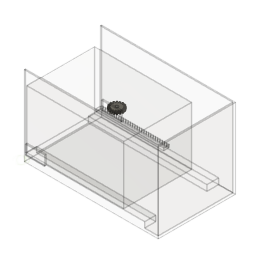
g25_gearmechanism_prototype (Autodesk Fusion 360 design; units mm, degrees)
part number: 2026-04-13-13-34-47-788
part number: 2026-04-13-16-24-35-810
part number: 2026-04-13-16-24-42-049
part number: 2026-04-13-16-24-44-900
Autodesk Fusion 360 part; units mm, degrees
sketch "AA_Sketch" plane through (0, 0, 0) normal (0, 0, 1) x (1, 0, 0)
  line L0 (0, 0) -> (283, 0)
  line L1 (283, 0) -> (283, 160)
  line L2 (283, 160) -> (0, 160)
  line L3 (0, 160) -> (0, 0)
  dimension "d1" = 283
  dimension "d2" = 160
  measures "d1" horizontal distance of L0.start L0.end
  measures "d2" vertical distance of L0.end L1.end
extrude "Extrude1" add sketch "AA_Sketch" along normal blind 165 makes body 1
shell "Shell1" thickness 3 removed faces 1 at (94.3333, 53.3333, 165) on bodies 1
sketch "Sketch2" plane through (0, 0, 3) normal (0, 0, 1) x (-1, 0, 0)
  line L0 (-3, -157) -> (-3, -3)
  line L1 (-3, -3) -> (-280, -3)
  line L2 (-280, -3) -> (-280, -157)
  line L3 (-280, -157) -> (-3, -157)
sketch "AA_Sketch (1)" plane through (0, 0, 0) normal (0, 0, 1) x (1, 0, 0)
  line L0 (0, 0) -> (200, 0)
  line L1 (200, 0) -> (200, 140)
  line L2 (200, 140) -> (0, 140)
  line L3 (0, 140) -> (0, 0)
  dimension "d6" = 200
  dimension "d7" = 140
  measures "d6" horizontal distance of L0.start L0.end
  measures "d7" vertical distance of L0.end L1.end
extrude "Extrude2" add sketch "AA_Sketch (1)" along normal blind 120 separate body makes body 2
move_body "Move1" bodies 2 to x (1, 0, 0) y (0, 1, 0) z (0, 0, 1) at (48.081, 9.2189, 0)
sketch "Sketch5" plane through (0, 3, 0) normal (0, 1, 0) x (-1, 0, 0)
  line L0 (-280, 3) -> (-3, 3)
  line L1 (-3, 3) -> (-3, 165)
  line L2 (-3, 165) -> (-280, 165)
  line L3 (-280, 165) -> (-280, 3)
sketch "AA_Sketch (2)" plane through (0, 0, 0) normal (0, 0, 1) x (1, 0, 0)
  line L0 (0, 0) -> (250, 0)
  line L1 (250, 0) -> (250, 5)
  line L2 (250, 5) -> (0, 5)
  line L3 (0, 5) -> (0, 0)
  dimension "d16" = 250
  dimension "d17" = 5
  measures "d16" horizontal distance of L0.start L0.end
  measures "d17" vertical distance of L0.end L1.end
sketch "AA_Sketch (2) (2)" plane through (0, 0, 0) normal (0, 0, 1) x (1, 0, 0)
  line L0 (0, 0) -> (250, 0)
  line L1 (250, 0) -> (250, 25)
  line L2 (250, 25) -> (0, 25)
  line L3 (0, 25) -> (0, 0)
  dimension "d10" = 250
  dimension "d11" = 25
  measures "d10" horizontal distance of L0.start L0.end
  measures "d11" vertical distance of L0.end L1.end
extrude "Extrude3" add sketch "AA_Sketch (2) (2)" along normal blind 7 separate body makes body 3
extrude "Extrude4" add 1 faces at (83.3333, 16.6667, 7) along direction (0, 0, 1) blind 7 on bodies 3 bodies 3
move_body "Move2" bodies 3 to x (1, 0, 0) y (0, 1, 0) z (0, 0, 1) at (1.9978, 0.899, 0.4525)
copy_body "CopyPasteBodies1" bodies 3 makes body 4
move_body "Move3" bodies 3 to x (1, 0, 0) y (0, 1, 0) z (0, 0, 1) at (-0.1358, 112.2274, 0)
move_body "Move4" bodies 3 to x (1, 0, 0) y (0, 1, 0) z (0, 0, 1) at (-1.6414, 34.1917, 0)
move_body "Move5" bodies 3 to x (1, 0, 0) y (0, 1, 0) z (0, 0, 1) at (0.433, 1.9595, 0)
move_face "MoveFace1" by (10.1391, 1.7367, 0) 1 faces at (83.9869, 165.9443, 14.4525) on bodies 3
move_body "Move6" bodies 2 to x (1, 0, 0) y (0, 1, 0) z (0, 0, 1) at (0, 1.2677, 9.5453)
move_body "Move7" bodies 2 to x (1, 0, 0) y (0, 1, 0) z (0, 0, 1) at (0, 0, 5.0574)
sketch "Base Circle" plane through (0, 0, 0) normal (0, 0, 1) x (1, 0, 0)
  circle A0 centre (0, 0) radius 10.2645
  circle A1 centre (0, 0) radius 3
extrude "Extrude6" add sketch "Base Circle" along normal blind 5 separate body makes body 5
sketch "Gear Tooth" plane through (0, 0, 0) normal (0, 0, 1) x (1, 0, 0)
  spline S0 degree 5 poles (11.2043, -1.2724) (11.2108, -1.2731) (11.2238, -1.2744) (11.2433, -1.2758) (11.2694, -1.2766) (11.3021, -1.2761) (11.3349, -1.2745) (11.3678, -1.2724) (11.4006, -1.2698) (11.4335, -1.267) (11.4664, -1.264) (11.4994, -1.2606) (11.5323, -1.2568) (11.5653, -1.2525) (11.5983, -1.2477) (11.6313, -1.2424) (11.6643, -1.2367) (11.6973, -1.2306) (11.7303, -1.2242) (11.7633, -1.2176) (11.7964, -1.2107) (11.8294, -1.2034) (11.8624, -1.1959) (11.8954, -1.188) (11.9285, -1.1798) (11.9615, -1.1713) (11.9945, -1.1625) (12.0275, -1.1534) (12.0605, -1.1441) (12.0935, -1.1345) (12.1265, -1.1246) (12.1594, -1.1145) (12.1924, -1.1041) (12.2253, -1.0934) (12.2583, -1.0825) (12.2912, -1.0713) (12.3241, -1.0599) (12.3569, -1.0482) (12.3898, -1.0363) (12.4226, -1.0241) (12.4555, -1.0117) (12.4883, -0.9991) (12.521, -0.9862) (12.5538, -0.9731) (12.5865, -0.9597) (12.6192, -0.9462) (12.6519, -0.9324) (12.6846, -0.9184) (12.7172, -0.9041) (12.7498, -0.8897) (12.7824, -0.875) (12.815, -0.8601) (12.8475, -0.845) (12.88, -0.8296) (12.9125, -0.8141) (12.9449, -0.7983) (12.9773, -0.7823) (13.0097, -0.7662) (13.042, -0.7498) (13.0743, -0.7332) (13.1066, -0.7164) (13.1388, -0.6994) (13.171, -0.6822) (13.2031, -0.6648) (13.2353, -0.6472) (13.2673, -0.6294) (13.2994, -0.6114) (13.3314, -0.5931) (13.3633, -0.5747) (13.3953, -0.5562) (13.4271, -0.5374) (13.4526, -0.5222) (13.4717, -0.5107) (13.4844, -0.503) (13.4908, -0.4992) knots 0 0 0 0 0 0 0.01428571 0.02857143 0.04285714 0.05714286 0.07142857 0.08571429 0.1 0.11428571 0.12857143 0.14285714 0.15714286 0.17142857 0.18571429 0.2 0.21428571 0.22857143 0.24285714 0.25714286 0.27142857 0.28571429 0.3 0.31428571 0.32857143 0.34285714 0.35714286 0.37142857 0.38571429 0.4 0.41428571 0.42857143 0.44285714 0.45714286 0.47142857 0.48571429 0.5 0.51428571 0.52857143 0.54285714 0.55714286 0.57142857 0.58571429 0.6 0.61428571 0.62857143 0.64285714 0.65714286 0.67142857 0.68571429 0.7 0.71428571 0.72857143 0.74285714 0.75714286 0.77142857 0.78571429 0.8 0.81428571 0.82857143 0.84285714 0.85714286 0.87142857 0.88571429 0.9 0.91428571 0.92857143 0.94285714 0.95714286 0.97142857 0.98571429 1 1 1 1 1 1
  spline S1 degree 5 poles (11.2043, 1.2724) (11.2108, 1.2731) (11.2238, 1.2744) (11.2433, 1.2758) (11.2694, 1.2766) (11.3021, 1.2761) (11.3349, 1.2745) (11.3678, 1.2724) (11.4006, 1.2698) (11.4335, 1.267) (11.4664, 1.264) (11.4994, 1.2606) (11.5323, 1.2568) (11.5653, 1.2525) (11.5983, 1.2477) (11.6313, 1.2424) (11.6643, 1.2367) (11.6973, 1.2306) (11.7303, 1.2242) (11.7633, 1.2176) (11.7964, 1.2107) (11.8294, 1.2034) (11.8624, 1.1959) (11.8954, 1.188) (11.9285, 1.1798) (11.9615, 1.1713) (11.9945, 1.1625) (12.0275, 1.1534) (12.0605, 1.1441) (12.0935, 1.1345) (12.1265, 1.1246) (12.1594, 1.1145) (12.1924, 1.1041) (12.2253, 1.0934) (12.2583, 1.0825) (12.2912, 1.0713) (12.3241, 1.0599) (12.3569, 1.0482) (12.3898, 1.0363) (12.4226, 1.0241) (12.4555, 1.0117) (12.4883, 0.9991) (12.521, 0.9862) (12.5538, 0.9731) (12.5865, 0.9597) (12.6192, 0.9462) (12.6519, 0.9324) (12.6846, 0.9184) (12.7172, 0.9041) (12.7498, 0.8897) (12.7824, 0.875) (12.815, 0.8601) (12.8475, 0.845) (12.88, 0.8296) (12.9125, 0.8141) (12.9449, 0.7983) (12.9773, 0.7823) (13.0097, 0.7662) (13.042, 0.7498) (13.0743, 0.7332) (13.1066, 0.7164) (13.1388, 0.6994) (13.171, 0.6822) (13.2031, 0.6648) (13.2353, 0.6472) (13.2673, 0.6294) (13.2994, 0.6114) (13.3314, 0.5931) (13.3633, 0.5747) (13.3953, 0.5562) (13.4271, 0.5374) (13.4526, 0.5222) (13.4717, 0.5107) (13.4844, 0.503) (13.4908, 0.4992) knots 0 0 0 0 0 0 0.01428571 0.02857143 0.04285714 0.05714286 0.07142857 0.08571429 0.1 0.11428571 0.12857143 0.14285714 0.15714286 0.17142857 0.18571429 0.2 0.21428571 0.22857143 0.24285714 0.25714286 0.27142857 0.28571429 0.3 0.31428571 0.32857143 0.34285714 0.35714286 0.37142857 0.38571429 0.4 0.41428571 0.42857143 0.44285714 0.45714286 0.47142857 0.48571429 0.5 0.51428571 0.52857143 0.54285714 0.55714286 0.57142857 0.58571429 0.6 0.61428571 0.62857143 0.64285714 0.65714286 0.67142857 0.68571429 0.7 0.71428571 0.72857143 0.74285714 0.75714286 0.77142857 0.78571429 0.8 0.81428571 0.82857143 0.84285714 0.85714286 0.87142857 0.88571429 0.9 0.91428571 0.92857143 0.94285714 0.95714286 0.97142857 0.98571429 1 1 1 1 1 1
  arc A0 (13.4908, -0.4992) -> (13.4908, 0.4992) centre (0, 0) ccw
  line L0 (10.189, -1.1571) -> (11.2043, -1.2724)
  line L1 (10.189, 1.1571) -> (11.2043, 1.2724)
  line L2 (10.189, -1.1571) -> (10.189, 1.1571)
  point P0 (11.3641, -1.2725)
  point P1 (11.5256, -1.2575)
  point P2 (11.688, -1.2323)
  point P3 (11.8512, -1.1984)
  point P4 (12.0149, -1.1569)
  point P5 (12.179, -1.1083)
  point P6 (12.3433, -1.053)
  point P7 (12.5078, -0.9914)
  point P8 (12.6722, -0.9237)
  point P9 (12.8365, -0.85)
  point P10 (13.0007, -0.7706)
  point P11 (13.1645, -0.6856)
  point P12 (13.3279, -0.5951)
  point P13 (11.3641, 1.2725)
  point P14 (11.5256, 1.2575)
  point P15 (11.688, 1.2323)
  point P16 (11.8512, 1.1984)
  point P17 (12.0149, 1.1569)
  point P18 (12.179, 1.1083)
  point P19 (12.3433, 1.053)
  point P20 (12.5078, 0.9914)
  point P21 (12.6722, 0.9237)
  point P22 (12.8365, 0.85)
  point P23 (13.0007, 0.7706)
  point P24 (13.1645, 0.6856)
  point P25 (13.3279, 0.5951)
extrude "Extrude7" add sketch "Gear Tooth" along normal blind 5 bodies 5
fillet "Fillet1" radius 0.5 2 edges at (10.1989, -1.1582, 2.5) (10.1989, 1.1582, 2.5) on bodies 5
pattern_circular "C-Pattern1" count 16 over 360 about axis through (0, 0, 0) along (0, 0, 1) of "Extrude7", "Fillet1"
sketch "Diametrial Pitch Circle" plane through (0, 0, 0) normal (0, 0, 1) x (1, 0, 0)
  circle A0 centre (0, 0) radius 12 construction
sketch "RackSketch" plane through (0, 0, 0) normal (0, 0, 1) x (1, 0, 0)
  line L0 (0, 0) -> (140, 0)
  line L1 (140, 0) -> (140, 25)
  line L2 (140, 25) -> (0, 25)
  line L3 (0, 25) -> (0, 0)
  line L4 (0, 10) -> (4.7, 13)
  line L5 (4.7, 13) -> (4.7, 10)
  line L6 (4.7, 10) -> (0, 10)
  dimension "d28" = 140
  dimension "d29" = 25
  dimension "d30" = 5.5758
  dimension "d31" = 3
  dimension "d32" = 4.7
  measures "d28" horizontal distance of L0.start L0.end
  measures "d29" vertical distance of L0.end L1.end
  measures "d30" distance of L4.start L4.end
  measures "d31" distance of L4.end L5.end
  measures "d32" distance of L5.end L4.start
sketch "RackProfile" plane through (0, 0, 0) normal (0, 0, 1) x (1, 0, 0)
  line L0 (0, 0) -> (140, 0)
  line L1 (140, 0) -> (140, 10)
  line L2 (140, 10) -> (0, 10)
  line L3 (0, 10) -> (0, 0)
  line L4 (0, 10) -> (2.35, 13)
  line L5 (2.35, 13) -> (4.7, 10)
  line L6 (4.7, 10) -> (7.05, 13)
  line L7 (7.05, 13) -> (9.4, 10)
  line L8 (9.4, 10) -> (11.75, 13)
  line L9 (11.75, 13) -> (14.1, 10)
  line L10 (14.1, 10) -> (16.45, 13)
  line L11 (16.45, 13) -> (18.8, 10)
  line L12 (18.8, 10) -> (21.15, 13)
  line L13 (21.15, 13) -> (23.5, 10)
  line L14 (23.5, 10) -> (25.85, 13)
  line L15 (25.85, 13) -> (28.2, 10)
  line L16 (28.2, 10) -> (30.55, 13)
  line L17 (30.55, 13) -> (32.9, 10)
  line L18 (32.9, 10) -> (35.25, 13)
  line L19 (35.25, 13) -> (37.6, 10)
  line L20 (37.6, 10) -> (39.95, 13)
  line L21 (39.95, 13) -> (42.3, 10)
  line L22 (42.3, 10) -> (44.65, 13)
  line L23 (44.65, 13) -> (47, 10)
  line L24 (47, 10) -> (49.35, 13)
  line L25 (49.35, 13) -> (51.7, 10)
  line L26 (51.7, 10) -> (54.05, 13)
  line L27 (54.05, 13) -> (56.4, 10)
  line L28 (56.4, 10) -> (58.75, 13)
  line L29 (58.75, 13) -> (61.1, 10)
  line L30 (61.1, 10) -> (63.45, 13)
  line L31 (63.45, 13) -> (65.8, 10)
  line L32 (65.8, 10) -> (68.15, 13)
  line L33 (68.15, 13) -> (70.5, 10)
  line L34 (70.5, 10) -> (72.85, 13)
  line L35 (72.85, 13) -> (75.2, 10)
  line L36 (75.2, 10) -> (77.55, 13)
  line L37 (77.55, 13) -> (79.9, 10)
  line L38 (79.9, 10) -> (82.25, 13)
  line L39 (82.25, 13) -> (84.6, 10)
  line L40 (84.6, 10) -> (86.95, 13)
  line L41 (86.95, 13) -> (89.3, 10)
  line L42 (89.3, 10) -> (91.65, 13)
  line L43 (91.65, 13) -> (94, 10)
  line L44 (94, 10) -> (96.35, 13)
  line L45 (96.35, 13) -> (98.7, 10)
  line L46 (98.7, 10) -> (101.05, 13)
  line L47 (101.05, 13) -> (103.4, 10)
  line L48 (103.4, 10) -> (105.75, 13)
  line L49 (105.75, 13) -> (108.1, 10)
  line L50 (108.1, 10) -> (110.45, 13)
  line L51 (110.45, 13) -> (112.8, 10)
  line L52 (112.8, 10) -> (115.15, 13)
  line L53 (115.15, 13) -> (117.5, 10)
  line L54 (117.5, 10) -> (119.85, 13)
  line L55 (119.85, 13) -> (122.2, 10)
  line L56 (122.2, 10) -> (124.55, 13)
  line L57 (124.55, 13) -> (126.9, 10)
  line L58 (126.9, 10) -> (129.25, 13)
  line L59 (129.25, 13) -> (131.6, 10)
  line L60 (131.6, 10) -> (133.95, 13)
  line L61 (133.95, 13) -> (136.3, 10)
  line L62 (136.3, 10) -> (138.65, 13)
  line L63 (138.65, 13) -> (140, 10)
  dimension "d91" = 140
  dimension "d92" = 10
  dimension "d93" = 3.8108
  dimension "d94" = 3.8108
  dimension "d95" = 3.8108
  dimension "d96" = 3.8108
  dimension "d97" = 3.8108
  dimension "d98" = 3.8108
  dimension "d99" = 3.8108
  dimension "d100" = 3.8108
  dimension "d101" = 3.8108
  dimension "d102" = 3.8108
  dimension "d103" = 3.8108
  dimension "d104" = 3.8108
  dimension "d105" = 3.8108
  dimension "d106" = 3.8108
  dimension "d107" = 3.8108
  dimension "d108" = 3.8108
  dimension "d109" = 3.8108
  dimension "d110" = 3.8108
  dimension "d111" = 3.8108
  dimension "d112" = 3.8108
  dimension "d113" = 3.8108
  dimension "d114" = 3.8108
  dimension "d115" = 3.8108
  dimension "d116" = 3.8108
  dimension "d117" = 3.8108
  dimension "d118" = 3.8108
  dimension "d119" = 3.8108
  dimension "d120" = 3.8108
  dimension "d121" = 3.8108
  dimension "d122" = 3.8108
  dimension "d123" = 3.8108
  dimension "d124" = 3.8108
  dimension "d125" = 3.8108
  dimension "d126" = 3.8108
  dimension "d127" = 3.8108
  dimension "d128" = 3.8108
  dimension "d129" = 3.8108
  dimension "d130" = 3.8108
  dimension "d131" = 3.8108
  dimension "d132" = 3.8108
  dimension "d133" = 3.8108
  dimension "d134" = 3.8108
  dimension "d135" = 3.8108
  dimension "d136" = 3.8108
  dimension "d137" = 3.8108
  dimension "d138" = 3.8108
  dimension "d139" = 3.8108
  dimension "d140" = 3.8108
  dimension "d141" = 3.8108
  dimension "d142" = 3.8108
  dimension "d143" = 3.8108
  dimension "d144" = 3.8108
  dimension "d145" = 3.8108
  dimension "d146" = 3.8108
  dimension "d147" = 3.8108
  dimension "d148" = 3.8108
  dimension "d149" = 3.8108
  dimension "d150" = 3.8108
  dimension "d151" = 3.8108
  dimension "d152" = 3.2898
  measures "d91" horizontal distance of L0.start L0.end
  measures "d92" vertical distance of L0.end L1.end
  measures "d93" distance of L2.end L4.end
  measures "d94" distance of L4.end L5.end
  measures "d95" distance of L5.end L6.end
  measures "d96" distance of L6.end L7.end
  measures "d97" distance of L7.end L8.end
  measures "d98" distance of L8.end L9.end
  measures "d99" distance of L9.end L10.end
  measures "d100" distance of L10.end L11.end
  measures "d101" distance of L11.end L12.end
  measures "d102" distance of L12.end L13.end
  measures "d103" distance of L13.end L14.end
  measures "d104" distance of L14.end L15.end
  measures "d105" distance of L15.end L16.end
  measures "d106" distance of L16.end L17.end
  measures "d107" distance of L17.end L18.end
  measures "d108" distance of L18.end L19.end
  measures "d109" distance of L19.end L20.end
  measures "d110" distance of L20.end L21.end
  measures "d111" distance of L21.end L22.end
  measures "d112" distance of L22.end L23.end
  measures "d113" distance of L23.end L24.end
  measures "d114" distance of L24.end L25.end
  measures "d115" distance of L25.end L26.end
  measures "d116" distance of L26.end L27.end
  measures "d117" distance of L27.end L28.end
  measures "d118" distance of L28.end L29.end
  measures "d119" distance of L29.end L30.end
  measures "d120" distance of L30.end L31.end
  measures "d121" distance of L31.end L32.end
  measures "d122" distance of L32.end L33.end
  measures "d123" distance of L33.end L34.end
  measures "d124" distance of L34.end L35.end
  measures "d125" distance of L35.end L36.end
  measures "d126" distance of L36.end L37.end
  measures "d127" distance of L37.end L38.end
  measures "d128" distance of L38.end L39.end
  measures "d129" distance of L39.end L40.end
  measures "d130" distance of L40.end L41.end
  measures "d131" distance of L41.end L42.end
  measures "d132" distance of L42.end L43.end
  measures "d133" distance of L43.end L44.end
  measures "d134" distance of L44.end L45.end
  measures "d135" distance of L45.end L46.end
  measures "d136" distance of L46.end L47.end
  measures "d137" distance of L47.end L48.end
  measures "d138" distance of L48.end L49.end
  measures "d139" distance of L49.end L50.end
  measures "d140" distance of L50.end L51.end
  measures "d141" distance of L51.end L52.end
  measures "d142" distance of L52.end L53.end
  measures "d143" distance of L53.end L54.end
  measures "d144" distance of L54.end L55.end
  measures "d145" distance of L55.end L56.end
  measures "d146" distance of L56.end L57.end
  measures "d147" distance of L57.end L58.end
  measures "d148" distance of L58.end L59.end
  measures "d149" distance of L59.end L60.end
  measures "d150" distance of L60.end L61.end
  measures "d151" distance of L61.end L62.end
  measures "d152" distance of L62.end L1.end
extrude "Extrude8" add sketch "RackProfile" along normal blind 5 separate body makes body 6
move_body "Move8" bodies 6 to x (1, 0, 0) y (0, 1, 0) z (0, 0, 1) at (50.6074, 152.1145, 19.3223)
combine "Combine1" operation add target body 6 tool bodies 2 makes body 7 at (114.7477, 57.1532, 14.6027)
combine "Combine2" operation add target body 7 tool bodies 6 makes body 8 at (120.7741, 155.4478, 19.3223)
move_body "Move9" bodies 8 to x (1, 0, 0) y (0, 1, 0) z (0, 0, 1) at (0, -1.8116, -0.0016)
combine "Combine3" operation add target body 8 tool bodies 7
move_body "Move10" bodies 5 to x (1, 0, 0) y (0, 1, 0) z (0, 0, 1) at (69.7672, 174.3212, 20.7438)
move_body "Move11" bodies 8 to x (1, 0, 0) y (0, 1, 0) z (0, 0, 1) at (0, -7.2492, 0.3052)
move_body "Move12" bodies 8 to x (1, 0, 0) y (0, 1, 0) z (0, 0, 1) at (0.2129, 1.799, 0)
move_body "Move13" bodies 8 to x (1, 0, 0) y (0, 1, 0) z (0, 0, 1) at (-40.6079, -1.0144, 0)
move_body "Move14" bodies 5 to x (1, 0, 0) y (0, 1, 0) z (0, 0, 1) at (-40.8763, -5.5836, 0)
sketch "GearHoleSketch" plane through (0, 160, 0) normal (0, 1, 0) x (-1, 0, 0)
  line L0 (-283, 0) -> (0, 0)
  line L1 (0, 0) -> (0, 165)
  line L2 (0, 165) -> (-283, 165)
  line L3 (-283, 165) -> (-283, 0)
  line L4 (-8.89, 13.24, -160) -> (-48.89, 13.24, -160)
  line L5 (-48.89, 13.24, -160) -> (-48.89, 33.24, -160)
  line L6 (-48.89, 33.24, -160) -> (-8.89, 33.24, -160)
  line L7 (-8.89, 33.24, -160) -> (-8.89, 13.24, -160)
  dimension "d172" = 40
  dimension "d173" = 20
extrude "Extrude11" cut sketch "GearHoleSketch" along normal through all contours L4 L5 L6 L7 in plane through (0, 0, 0) normal (0, 1, 0) bodies 1
move_body "Move15" bodies 3 to x (1, 0, 0) y (0, 1, 0) z (0, 0, 1) at (0, -13.5908, -2.2656)
move_body "Move16" bodies 3 to x (1, 0, 0) y (0, 1, 0) z (0, 0, 1) at (0, -2.8348, 2.8286)
combine "Combine4" operation add target body 4 tool bodies 1
combine "Combine5" operation add target body 3 tool bodies 4
sketch "Sketch20" plane through (0, 0, 0) normal (-1, 0, 0) x (0, -1, 0)
  line L0 (-160, 0) -> (0, 0)
  line L1 (0, 0) -> (0, 165)
  line L2 (0, 165) -> (-160, 165)
  line L3 (-160, 165) -> (-160, 0)
  line L4 (-160, 165) -> (0, 165)
  line L5 (0, 165) -> (0, 0)
  line L6 (0, 0) -> (-160, 0)
  line L7 (-160, 0) -> (-160, 165)
  constraint horizontal L4
  constraint vertical L5
  constraint horizontal L6
  constraint vertical L7
  constraint coincident L0.end L1.start
  constraint coincident L2.end L3.start
extrude "Extrude12" cut sketch "Sketch20" against normal blind 6 bodies 3
copy_body "Body->Comp1" bodies 3 removing the originals makes body 9 in component "Component"
copy_body "Body->Comp2" bodies 5 removing the originals makes body 10 in component "Spur Gear (16 teeth)"
copy_body "Body->Comp3" bodies 8 removing the originals makes body 11 in component "Component'"
sketch "AA_Sketch (3)" plane through (0, 0, 0) normal (0, 0, 1) x (1, 0, 0) in component "Spur Gear (16 teeth)"
sketch "Sketch2 (2)" plane through (0, 0, 0) normal (1, 0, 0) x (0, 1, 0) in component "Spur Gear (16 teeth)"
  line L0 (160, -10) -> (150, -10)
  line L1 (150, -10) -> (150, -20)
  line L2 (150, -20) -> (160, -20)
  line L3 (160, -20) -> (160, -10)
  constraint horizontal L0
  constraint vertical L1
  constraint horizontal L2
  constraint vertical L3
component "Component" placed x (1, 0, 0) y (0, 1, 0) z (0, 0, 1) at (0, 0, 0)
component "Spur Gear (16 teeth)" placed x (1, 0, 0) y (0, 1, 0) z (0, 0, 1) at (0, 0, 0)
component "Component'" placed x (1, 0, 0) y (0, 1, 0) z (0, 0, 1) at (0, 0, 0)
named bodies: "Spur Gear (16 teeth)"
